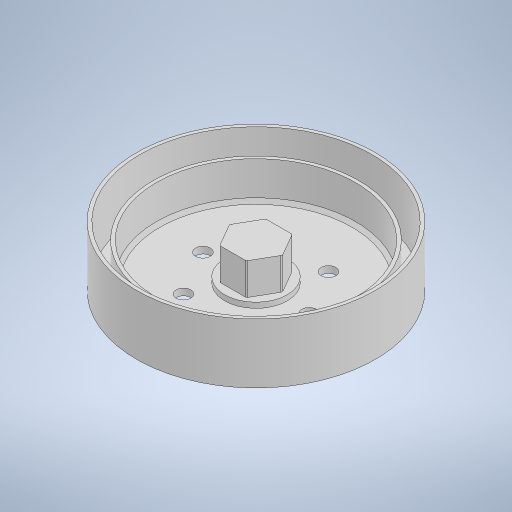
# Autodesk Inventor part: Wheel V2 Mold
Saved by Autodesk Inventor 2023.2 (Build 272271000, 271)
## iProperties
Created: 2023-06-08
Part Number: Wheel V2 Mold
Material: Generic
Document SubType Name: Modeling
Designer: Nathan Cai
Density: 1 g/cm^3
Appearance: Default
Author: Nathan Cai
Autodesk Inventor part; units mm, degrees
ref_plane "YZ Plane" through (0, 0, 0) normal (1, 0, 0) x (0, 1, 0)
ref_plane "XZ Plane" through (0, 0, 0) normal (0, 1, 0) x (-1, 0, 0)
ref_plane "XY Plane" through (0, 0, 0) normal (0, 0, 1) x (1, 0, 0)
sketch "Sketch1" plane through (0, 0, 0) normal (0, 1, 0) x (-1, 0, 0)
  circle A0 centre (0, 0) radius 28.575
  dimension "d0" = 57.15
  constraints: 1 centre point, 1 coincident
  measures "d0" diameter of A0
extrude "Extrusion1" add sketch "Sketch1" along normal blind 1.5875
sketch "Sketch2" plane through (0, 1.5875, 0) normal (0, 1, 0) x (1, 0, 0)
  line L0 (0, 0) -> (-28.575, 0) construction
  circle A0 centre (0, 0) radius 28.575 projected
  line L1 (-6.35, 0) -> (-3.175, 5.4993)
  line L2 (-3.175, 5.4993) -> (3.175, 5.4993)
  line L3 (3.175, 5.4993) -> (6.35, 0)
  line L4 (6.35, 0) -> (3.175, -5.4993)
  line L5 (3.175, -5.4993) -> (-3.175, -5.4993)
  line L6 (-3.175, -5.4993) -> (-6.35, 0)
  circle A1 centre (0, 0) radius 23.8125
  circle A2 centre (0, 0) radius 24.6063
  circle A3 centre (0, 0) radius 27.7812
  circle A4 centre (0, 0) radius 7.493
  circle A5 centre (0, 0) radius 12.7 construction
  circle A6 centre (-12.7, 0) radius 1.7526
  circle A7 centre (-6.35, -10.9985) radius 1.7526
  circle A8 centre (6.35, -10.9985) radius 1.7526
  circle A9 centre (12.7, 0) radius 1.7526
  circle A10 centre (6.35, 10.9985) radius 1.7526
  circle A11 centre (-6.35, 10.9985) radius 1.7526
  dimension "d18" = 25.4
  dimension "d3" = 6.35
  dimension "d4" = 47.625
  dimension "d5" = 0.7937
  dimension "d6" = 0.7937
  dimension "d15" = 14.986
  dimension "d19" = 3.5052
  dimension "d22" = 360
  constraints: 14 end point, 10 centre point, 5 coincident, 2 horizontal alignment, 2 point on line, 1 horizontal, 29 other
  measures "d3" distance of L0.start L1.start
  measures "d4" diameter of A1
  measures "d5" radial gap between concentric circles of A1 A2
  measures "d15" diameter of A4
  measures "d19" diameter of A6
extrude "Extrusion2" add sketch "Sketch2" along normal blind 8.89 contours L1 L2 L3 L4 L5 L6 | A2
fillet "Fillet1" radius 0.508 6 edges at (6.35, 6.0325, 0) (3.175, 6.0325, -5.4993) (-3.175, 6.0325, -5.4993) (-6.35, 6.0325, 0) (-3.175, 6.0325, 5.4993) (3.175, 6.0325, 5.4993)
extrude "Extrusion3" add sketch "Sketch2" along normal blind 12.7 contours A0
chamfer "Chamfer1" distance 0.7937 angle 45 1 edges at (-23.8125, 1.5875, 0)
extrude "Extrusion4" add sketch "Sketch2" along normal blind 1.27 contours L1 L2 L3 L4 L5 L6 | A4
extrude "Extrusion5" cut sketch "Sketch2" against normal through all contours A6 | A7 | A8 | A9 | A10 | A11
body "Solid1"
